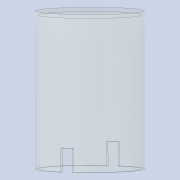
# Autodesk Inventor part: Part6_containter_top
Saved by Autodesk Inventor 2020 (Build 240168000, 168)
## iProperties
Created: 2019-07-03
Part Number: Part6_containter_top
Material: ABS Plastic
Document SubType Name: Modeling
Designer: kimhos
Density: 1.06 g/cm^3
Appearance: Clear - Light
Author: kimhos
Autodesk Inventor part; units mm, degrees
ref_plane "YZ Plane" through (0, 0, 0) normal (1, 0, 0) x (0, 1, 0)
ref_plane "XZ Plane" through (0, 0, 0) normal (0, 1, 0) x (-1, 0, 0)
ref_plane "XY Plane" through (0, 0, 0) normal (0, 0, 1) x (1, 0, 0)
sketch "Sketch2" plane through (0, 0, 0) normal (0, 1, 0) x (-1, 0, 0)
  circle A0 centre (0, 0) radius 13.8
  line L0 (0, -13.8) -> (0, -13)
  dimension "d0" = 27.6
  dimension "d79" = 0.8
  constraints: 2 end point, 1 coincident, 1 vertical, 1 vertical alignment, 2 other
  measures "d79" distance of L0.start L0.end
extrude "Extrusion1" add sketch "Sketch2" along normal blind 40
sketch "Sketch3" plane through (0, 40, 0) normal (0, 1, 0) x (1, 0, 0)
  circle A0 centre (0, 0) radius 13
  dimension "d3" = 26
  constraints: 1 centre point, 1 coincident
  measures "d3" diameter of A0
hole "Hole1" at (0, 40, 0) direction (0, -1, 0) diameter 26 depth 39
sketch "Sketch8" plane through (0, 40, 0) normal (0, 1, 0) x (1, 0, 0)
  circle A0 centre (0, 0) radius 13.8 projected
  line L0 (-13.8, 0) -> (-13.8, 1.6)
  line L1 (-13.8, 0) -> (-12.2, 0) construction
  line L2 (-13.8, 1.6) -> (-10.8, 1.6)
  line L3 (-10.8, 1.6) -> (-10.8, -1.6)
  line L4 (-10.8, -1.6) -> (-13.8, -1.6)
  line L5 (-13.8, -1.6) -> (-13.8, 0)
  point P0 (-13.7069, 1.6)
  point P1 (-13.7069, -1.6)
  dimension "d64" = 1.6
  dimension "d66" = 3
  dimension "d67" = 3.2
  dimension "d69" = 3
  constraints: 12 end point, 3 perpendicular, 2 horizontal, 2 vertical, 2 other
  measures "d64" distance of L0.start L0.end
  measures "d66" distance of L0.end L2.end
  measures "d67" distance of L2.end L3.end
  measures "d69" distance of L3.end L4.end
extrude "Extrusion6" cut sketch "Sketch8" against normal blind 6.1 contours L2 L3 L4 A0 picked at (-11.8, 0)
sketch "Sketch9" plane through (0, 40, 0) normal (0, 1, 0) x (1, 0, 0)
  circle A0 centre (0, 0) radius 13.8 projected
  line L0 (13.8, 0) -> (13.8, 1.6)
  line L1 (13.8, 0) -> (15.4, 0) construction
  line L2 (13.8, 1.6) -> (10.8, 1.6)
  line L3 (10.8, 1.6) -> (10.8, -1.6)
  line L4 (10.8, -1.6) -> (13.8, -1.6)
  line L5 (13.8, -1.6) -> (13.8, 0)
  point P0 (13.7069, -1.6)
  point P1 (13.7069, 1.6)
  dimension "d72" = 1.6
  dimension "d74" = 3
  dimension "d75" = 3.2
  dimension "d76" = 3
  constraints: 12 end point, 3 perpendicular, 3 vertical, 1 horizontal, 1 point on line, 2 other
  measures "d72" distance of L0.start L0.end
  measures "d74" distance of L0.end L2.end
  measures "d75" distance of L2.end L3.end
  measures "d76" distance of L3.end L4.end
extrude "Extrusion7" cut sketch "Sketch9" against normal blind 6.1 contours A0 L4 L3 L2 picked at (11.8, 0)
body "Solid1"
